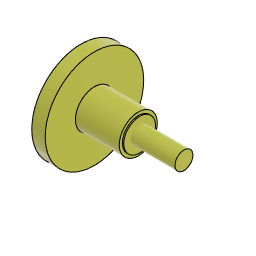
Boring Extruder v7 (Autodesk Fusion 360 archive; units mm, degrees)
design "LGX Primary Double Gear (reference dia)"
Autodesk Fusion 360 part; units mm, degrees
sketch "Sketch1" plane through (0, 0, 0) normal (1, 0, 0) x (0, 1, 0) in component "LGX Primary Double Gear"
  circle A0 centre (0, 0) radius 3.55
  circle A1 centre (0, 0) radius 11
  circle A2 centre (0, 0) radius 4.25
  circle A3 centre (0, 0) radius 2
  dimension "d3" = 7.1
  dimension "d24" = 22
  dimension "d25" = 8.5
  dimension "d26" = 4
  constraint coincident A0.centre A1.centre
  constraint concentric A1 A2
  constraint concentric A2 A3
  measures "d3" diameter of A0
  measures "d24" diameter of A1
  measures "d25" diameter of A2
  measures "d26" diameter of A3
extrude "Extrude1" add sketch "Sketch1" along normal blind 3 contours A1 makes body 1 in component "LGX Primary Double Gear"
extrude "Extrude2" add sketch "Sketch1" against normal blind 0.3 separate body contours A0 | A3 makes body 2 in component "LGX Primary Double Gear"
extrude "Extrude3" add sketch "Sketch1" along normal blind 13.4 from surface at -0.3 contours A0 | A3 bodies 2 in component "LGX Primary Double Gear"
extrude "Extrude4" add sketch "Sketch1" along normal up to surface (12.8 mm away) contours A2 bodies 1 2 in component "LGX Primary Double Gear"
extrude "Extrude1'" add sketch "Sketch1" along normal blind 23 and the other way blind 2 separate body contours A3 makes body 3 in component "LGX Primary Double Gear"
component "LGX Primary Double Gear" placed x (1, 0, 0) y (0, 1, 0) z (0, 0, 1) at (0, 0, 0)
named bodies: "Body1 (1)"

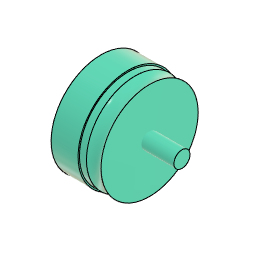
design "LGX Drive Gear (reference dia)"
Autodesk Fusion 360 part; units mm, degrees
sketch "Sketch1" plane through (0, 0, 0) normal (1, 0, 0) x (0, 1, 0) in component "LGX Drive Gear (reference dia)"
  circle A0 centre (0, 0) radius 9.25
  circle A1 centre (0, 0) radius 9
  circle A2 centre (0, 0) radius 1.5
  dimension "d1" = 18.5
  dimension "d2" = 18
  dimension "d10" = 3
  constraint coincident A0.centre A1.centre
  constraint concentric A0 A2
  measures "d1" diameter of A0
  measures "d2" diameter of A1
  measures "d10" diameter of A2
extrude "Extrude1" add sketch "Sketch1" against normal blind 5 contours A0 | A1 | A2 makes body 1 in component "LGX Drive Gear (reference dia)"
extrude "Extrude2" add sketch "Sketch1" along normal blind 4 separate body contours A1 | A2 makes body 2 in component "LGX Drive Gear (reference dia)"
sketch "Sketch2" plane through (0, 0, 0) normal (0, 1, 0) x (1, 0, 0) in component "LGX Drive Gear (reference dia)"
  line L0 (4, -9) -> (4, 9)
  line L1 (0, -9) -> (1.3, -9)
  arc A0 (4, -9) -> (1.3, -9) centre (2.65, -11.1042) ccw
  line L2 (1.3, -9) -> (4, -9)
  line L3 (0, -9) -> (0, 9)
  dimension "d7" = 1.3
  dimension "d8" = 2.5
  constraint coincident L0.start A0.start
  constraint horizontal L1
  constraint coincident L1.start L3.start
  measures "d7" distance of L1.start L1.end
  measures "d8" radius of A0
revolve "Revolve1" cut sketch "Sketch2" angle 360 about axis through (1.75, 0, 0) along (1, 0, 0) bodies 2 in component "LGX Drive Gear (reference dia)"
extrude "Extrude1'" add sketch "Sketch1" along normal mid plane 20 separate body contours A2 makes body 3 in component "LGX Drive Gear (reference dia)"
component "LGX Drive Gear (reference dia)" placed x (1, 0, 0) y (0, 1, 0) z (0, 0, 1) at (0, 0, 0)
named bodies: "Pinion", "Filament Driver"
